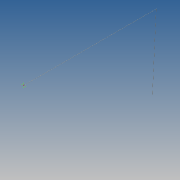
# Autodesk Inventor part: 2p2kfs
Saved by Autodesk Inventor 2014 SP1 (Build 180222100, 222)
## iProperties
Company: HERA Project
Created: 2013-05-28
Part Number: 2p2kfs
Material: Polyethylene, High Density
Document SubType Name: Modeling
Designer: David DeBoer
Density: 1 g/cm^3
Description: Kevlar feed support
Appearance: Smooth - Off-White
Author: David DeBoer
Title: Kevlar central support
Autodesk Inventor part; units mm, degrees
ref_plane "YZ Plane" through (0, 0, 0) normal (1, 0, 0) x (0, 1, 0)
ref_plane "XZ Plane" through (0, 0, 0) normal (0, 1, 0) x (-1, 0, 0)
ref_plane "XY Plane" through (0, 0, 0) normal (0, 0, 1) x (1, 0, 0)
sketch "Sketch1" plane through (0, 0, 0) normal (0, 0, 1) x (1, 0, 0)
  circle A0 centre (0, 0) radius 3.81
  dimension "d0" = 7.62
  constraints: 1 centre point, 1 coincident
  measures "d0" diameter of A0
extrude "Extrusion1" add sketch "Sketch1" along normal blind 8001
sketch "Sketch2" plane through (0, 0, 8001) normal (0, 0, 1) x (1, 0, 0)
  circle A0 centre (0, 0) radius 3.81 projected
  point P0 (0, 3.81)
  constraints: 1 vertical alignment, 1 other
ref_plane "Work Plane1" through (0, 3.81, 8001) normal (0, 1, 0) x (-1, 0, 0)
sketch "Sketch5" plane through (0, 3.81, 8001) normal (0, 1, 0) x (-1, 0, 0)
  line L0 (0, -8001) -> (3.81, -8001) construction
  dimension "d11" = 3.81
  constraints: 2 end point, 1 horizontal
  measures "d11" distance of L0.start L0.end
ref_plane "Work Plane2" through (0, 3.81, 0) normal (0, 0.9986295, -0.052336) x (-1, 0, 0)
sketch "Sketch6" plane through (0, 3.81, 0) normal (0, 0.9986295, -0.052336) x (-1, 0, 0)
  circle A0 centre (0, -0.1994) radius 3.81
  dimension "d13" = 7.62
  constraints: 1 centre point, 1 coincident
  measures "d13" diameter of A0
extrude "Extrusion4" add sketch "Sketch6" against normal blind 4495.8
body "Solid1"
